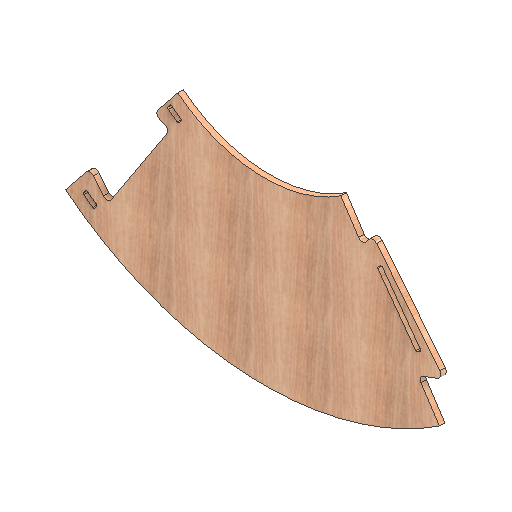
# Autodesk Inventor part: Platform F2
Saved by Autodesk Inventor 2021 (Build 250183000, 183)
## iProperties
Created: 2020-05-09
Part Number: Platform F2
Material: Wood (Birch)
Document SubType Name: Modeling
Designer: Dan Wikman
Density: 0.55 g/cm^3
Appearance: Birch - Natural Polished
Mass: 5289.03 g
Surface Area: 11405 cm^2
Volume: 9616.42 cm^3
Autodesk Inventor part; units mm, degrees
ref_plane "YZ Plane" through (0, 0, 0) normal (1, 0, 0) x (0, 1, 0)
ref_plane "XZ Plane" through (0, 0, 0) normal (0, 1, 0) x (-1, 0, 0)
ref_plane "XY Plane" through (0, 0, 0) normal (0, 0, 1) x (1, 0, 0)
sketch "CONTOURS" plane through (0, 0, 0) normal (0, 0, 1) x (1, 0, 0)
  arc A0 (968.4099, 588.6901) -> (991.7977, 587.5257) centre (980.5291, 596.6509) ccw
  line L0 (991.7977, 587.5257) -> (1002.4941, 600.7346)
  arc A1 (1026.6246, 600.6862) -> (1002.4941, 600.7346) centre (1014.5398, 590.9802) ccw
  line L1 (1026.6246, 600.6862) -> (1231.1426, 346.0447)
  arc A2 (1224.6125, 321.8682) -> (1231.1426, 346.0447) centre (1219.0578, 336.3387) ccw
  line L2 (1224.6125, 321.8682) -> (1176.7826, 303.508)
  arc A3 (1176.7826, 303.508) -> (1169.8597, 282.0103) centre (1181.9789, 289.9711) ccw
  line L3 (1169.8597, 282.0103) -> (1229.843, 190.694)
  arc A4 (19.8845, 247.8283) -> (1229.843, 190.694) centre (664.2228, 1052.783) ccw
  line L4 (19.8845, 247.8283) -> (87.3645, 332.0567)
  arc A5 (109.9494, 332.1158) -> (87.3645, 332.0567) centre (98.6808, 322.9907) ccw
  line L5 (109.9494, 332.1158) -> (142.2724, 292.2002)
  arc A6 (142.2724, 292.2002) -> (167.2836, 293.4607) centre (154.3182, 301.9547) ccw
  line L6 (167.2836, 293.4607) -> (347.6931, 568.841)
  arc A7 (347.6931, 568.841) -> (340.2824, 591.8055) centre (334.7277, 577.335) ccw
  line L7 (340.2824, 591.8055) -> (324.5349, 597.8504)
  arc A8 (318.415, 620.4534) -> (324.5349, 597.8504) centre (329.7312, 611.3873) ccw
  line L8 (318.415, 620.4534) -> (383.1767, 701.2887)
  arc A9 (383.1767, 701.2887) -> (910.792, 676.4054) centre (664.1546, 1052.9191) ccw
  line L9 (910.792, 676.4054) -> (968.4099, 588.6901)
  constraints: 20 end point, 20 point on circle, 10 centre point
sketch "HOLES" plane through (0, 0, 0) normal (0, 0, 1) x (1, 0, 0)
  arc A0 (351.3365, 645.2033) -> (352.2215, 639.6161) centre (354.5726, 642.8522) ccw
  line L0 (120.1263, 252.1125) -> (113.6606, 243.2133)
  arc A1 (108.0734, 242.3283) -> (113.6606, 243.2133) centre (110.4246, 245.5644) ccw
  line L1 (108.0734, 242.3283) -> (78.9488, 263.4886)
  arc A2 (78.0639, 269.0758) -> (78.9488, 263.4886) centre (81.3, 266.7247) ccw
  line L2 (78.0639, 269.0758) -> (84.5295, 277.975)
  arc A3 (90.1167, 278.8599) -> (84.5295, 277.975) centre (87.7656, 275.6239) ccw
  line L3 (90.1167, 278.8599) -> (119.2414, 257.6997)
  arc A4 (120.1263, 252.1125) -> (119.2414, 257.6997) centre (116.8902, 254.4636) ccw
  line L4 (381.3461, 618.4559) -> (352.2215, 639.6161)
  line L5 (351.3365, 645.2033) -> (357.8022, 654.1025)
  arc A5 (363.3894, 654.9874) -> (357.8022, 654.1025) centre (361.0382, 651.7514) ccw
  line L6 (363.3894, 654.9874) -> (392.514, 633.8272)
  arc A6 (393.3989, 628.24) -> (392.514, 633.8272) centre (390.1628, 630.5911) ccw
  line L7 (393.3989, 628.24) -> (386.9333, 619.3408)
  arc A7 (381.3461, 618.4559) -> (386.9333, 619.3408) centre (383.6972, 621.6919) ccw
  line L8 (1031.2196, 538.2098) -> (1040.1188, 544.6754)
  arc A8 (1045.706, 543.7905) -> (1040.1188, 544.6754) centre (1042.47, 541.4393) ccw
  line L9 (1045.706, 543.7905) -> (1168.5531, 374.7059)
  arc A9 (1167.6682, 369.1187) -> (1168.5531, 374.7059) centre (1165.3171, 372.3548) ccw
  line L10 (1167.6682, 369.1187) -> (1158.769, 362.6531)
  arc A10 (1153.1818, 363.538) -> (1158.769, 362.6531) centre (1156.4179, 365.8891) ccw
  line L11 (1153.1818, 363.538) -> (1030.3347, 532.6226)
  arc A11 (1031.2196, 538.2098) -> (1030.3347, 532.6226) centre (1033.5708, 534.9737) ccw
  constraints: 24 end point, 24 point on circle, 12 centre point
sketch "LETTERS" plane through (0, 0, 0) normal (0, 0, 1) x (1, 0, 0)
  line L0 (330.7596, 399.6732) -> (317.8052, 406.5947)
  line L1 (317.8052, 406.5947) -> (313.241, 398.0522)
  line L2 (313.241, 398.0522) -> (308.4708, 389.1241)
  line L3 (313.2079, 398.0531) -> (322.6164, 393.0261)
  constraints: 8 end point, 1 parallel, 1 perpendicular
extrude "Extrusion1" add sketch "CONTOURS" along normal blind 18
extrude "Extrusion2" cut sketch "HOLES" along normal blind 18
body "Solid1"
